Autodesk Inventor part; units mm, degrees
(part 2 of 2)
  arc A490 (63.341, 28.73) -> (62.579, 28.73) centre (62.96, 28.73) ccw
  arc A491 (65.119, 28.73) -> (65.881, 28.73) centre (65.5, 28.73) ccw
  arc A492 (65.881, 28.73) -> (65.119, 28.73) centre (65.5, 28.73) ccw
  arc A493 (65.119, 28.73) -> (65.881, 28.73) centre (65.5, 28.73) ccw
  arc A494 (65.881, 28.73) -> (65.119, 28.73) centre (65.5, 28.73) ccw
  arc A495 (67.659, 28.73) -> (68.421, 28.73) centre (68.04, 28.73) ccw
  arc A496 (68.421, 28.73) -> (67.659, 28.73) centre (68.04, 28.73) ccw
  arc A497 (67.659, 28.73) -> (68.421, 28.73) centre (68.04, 28.73) ccw
  arc A498 (68.421, 28.73) -> (67.659, 28.73) centre (68.04, 28.73) ccw
  arc A499 (70.199, 28.73) -> (70.961, 28.73) centre (70.58, 28.73) ccw
  arc A500 (70.961, 28.73) -> (70.199, 28.73) centre (70.58, 28.73) ccw
  arc A501 (70.199, 28.73) -> (70.961, 28.73) centre (70.58, 28.73) ccw
  arc A502 (70.961, 28.73) -> (70.199, 28.73) centre (70.58, 28.73) ccw
  arc A503 (72.739, 28.73) -> (73.501, 28.73) centre (73.12, 28.73) ccw
  arc A504 (73.501, 28.73) -> (72.739, 28.73) centre (73.12, 28.73) ccw
  arc A505 (72.739, 28.73) -> (73.501, 28.73) centre (73.12, 28.73) ccw
  arc A506 (73.501, 28.73) -> (72.739, 28.73) centre (73.12, 28.73) ccw
  arc A507 (75.279, 28.73) -> (76.041, 28.73) centre (75.66, 28.73) ccw
  arc A508 (76.041, 28.73) -> (75.279, 28.73) centre (75.66, 28.73) ccw
  arc A509 (75.279, 28.73) -> (76.041, 28.73) centre (75.66, 28.73) ccw
  arc A510 (76.041, 28.73) -> (75.279, 28.73) centre (75.66, 28.73) ccw
  arc A511 (77.819, 28.73) -> (78.581, 28.73) centre (78.2, 28.73) ccw
  arc A512 (78.581, 28.73) -> (77.819, 28.73) centre (78.2, 28.73) ccw
  arc A513 (77.819, 28.73) -> (78.581, 28.73) centre (78.2, 28.73) ccw
  arc A514 (78.581, 28.73) -> (77.819, 28.73) centre (78.2, 28.73) ccw
  arc A515 (89.59, 30.6) -> (89.59, 29.7) centre (89.59, 30.15) ccw
  arc A516 (89.59, 29.7) -> (89.59, 30.6) centre (89.59, 30.15) ccw
  arc A517 (89.59, 30.6) -> (89.59, 29.7) centre (89.59, 30.15) ccw
  arc A518 (89.59, 29.7) -> (89.59, 30.6) centre (89.59, 30.15) ccw
  arc A519 (87.05, 30.6) -> (87.05, 29.7) centre (87.05, 30.15) ccw
  arc A520 (87.05, 29.7) -> (87.05, 30.6) centre (87.05, 30.15) ccw
  arc A521 (87.05, 30.6) -> (87.05, 29.7) centre (87.05, 30.15) ccw
  arc A522 (87.05, 29.7) -> (87.05, 30.6) centre (87.05, 30.15) ccw
  arc A523 (84.51, 30.6) -> (84.51, 29.7) centre (84.51, 30.15) ccw
  arc A524 (84.51, 29.7) -> (84.51, 30.6) centre (84.51, 30.15) ccw
  arc A525 (84.51, 30.6) -> (84.51, 29.7) centre (84.51, 30.15) ccw
  arc A526 (84.51, 29.7) -> (84.51, 30.6) centre (84.51, 30.15) ccw
  line L251 (44.7388, 33.8709) -> (94, 33.8709)
  line L252 (94, 33.8709) -> (94, 24.2027)
  line L253 (94, 24.2027) -> (44.7388, 24.2027)
  line L254 (44.7388, 24.2027) -> (44.7388, 33.8709)
  line L255 (28.3727, 38.1472) -> (43.5417, 38.1472)
  line L256 (43.5417, 38.1472) -> (43.5417, 25.8726)
  line L257 (43.5417, 25.8726) -> (28.3727, 25.8726)
  line L258 (28.3727, 25.8726) -> (28.3727, 38.1472)
  line L259 (0, 194.7239) -> (130, 194.7239)
  line L260 (130, 194.7239) -> (130, 0)
  line L261 (130, 0) -> (0, 0)
  line L262 (0, 0) -> (0, 194.7239)
  circle A527 centre (65, 97.362) radius 8
  arc A528 (69.6765, 160.0343) -> (60.3235, 160.0343) centre (65, 167.7239) ccw
  line L263 (74.3631, 160.0343) -> (74.3631, 147.2613)
  line L264 (74.3631, 147.2613) -> (42.3354, 147.2613)
  line L265 (42.3354, 147.2613) -> (42.3354, 160.0343)
  line L266 (78, 180.9909) -> (100.5174, 180.9909)
  line L267 (100.5174, 180.9909) -> (100.5174, 168.379)
  line L268 (100.5174, 168.379) -> (78, 168.379)
  line L269 (78, 168.379) -> (78, 180.9909)
  line L270 (28.3727, 38.1472) -> (43.5417, 38.1472)
  line L271 (43.5417, 38.1472) -> (43.5417, 25.8726)
  line L272 (43.5417, 25.8726) -> (28.3727, 25.8726)
  line L273 (28.3727, 25.8726) -> (28.3727, 38.1472)
  line L274 (44.7388, 33.8709) -> (94, 33.8709)
  line L275 (94, 33.8709) -> (94, 24.2027)
  line L276 (94, 24.2027) -> (44.7388, 24.2027)
  line L277 (44.7388, 24.2027) -> (44.7388, 33.8709)
  circle A529 centre (45.5, 82.362) radius 1.6
  circle A530 centre (55.5, 82.362) radius 1.6
  circle A531 centre (65.5, 82.362) radius 1.6
  circle A532 centre (75.5, 82.362) radius 1.6
  circle A533 centre (85.5, 82.362) radius 1.6
  circle A534 centre (95.5, 82.362) radius 1.6
  circle A535 centre (45.5, 52.362) radius 1.6
  circle A536 centre (55.5, 52.362) radius 1.6
  circle A537 centre (65.5, 52.362) radius 1.6
  circle A538 centre (75.5, 52.362) radius 1.6
  circle A539 centre (85.5, 52.362) radius 1.6
  circle A540 centre (95.5, 52.362) radius 1.6
  circle A541 centre (34.5, 112.362) radius 1.6
  circle A542 centre (44.5, 112.362) radius 1.6
  circle A543 centre (54.5, 112.362) radius 1.6
  circle A544 centre (64.5, 112.362) radius 1.6
  circle A545 centre (74.5, 112.362) radius 1.6
  circle A546 centre (84.5, 112.362) radius 1.6
  circle A547 centre (34.5, 142.362) radius 1.6
  circle A548 centre (44.5, 142.362) radius 1.6
  circle A549 centre (54.5, 142.362) radius 1.6
  circle A550 centre (64.5, 142.362) radius 1.6
  circle A551 centre (74.5, 142.362) radius 1.6
  circle A552 centre (84.5, 142.362) radius 1.6
  circle A553 centre (38, 186.7239) radius 2.15
  circle A554 centre (52, 186.7239) radius 2.15
  circle A555 centre (78, 186.7239) radius 2.15
  circle A556 centre (92, 186.7239) radius 2.15
  circle A557 centre (38, 8) radius 2.15
  circle A558 centre (52, 8) radius 2.15
  circle A559 centre (78, 8) radius 2.15
  circle A560 centre (92, 8) radius 2.15
  circle A561 centre (8, 186.7239) radius 1.6
  circle A562 centre (122, 186.7239) radius 1.6
  circle A563 centre (122, 147.7239) radius 1.6
  circle A564 centre (122, 8) radius 1.6
  circle A565 centre (8, 8) radius 1.6
  line L278 (42.3354, 160.0343) -> (60.3235, 160.0343)
  line L279 (69.6765, 160.0343) -> (74.3631, 160.0343)
  point P0 (0, 0)
  constraints: 980 point on circle, 566 centre point, 560 end point, 40 coincident, 37 concentric, 20 parallel, 11 horizontal, 11 perpendicular, 2 point on line
sketch "スケッチ2" plane through (0, 0, 0) normal (0, 0, 1) x (1, 0, 0)
  point P0 (0, 0)
extrude "押し出し1" add sketch "スケッチ1" along normal blind 5.5 contours L3 L5 A32 L4 A17 A11 L251 L254 L253 L0 | L4 L253 L252 L251 A11 A17 A32 L5 L1 L0 | L3 L2 L4 A33 L58 L53 L52 A23 A29 A32 L5 | L5 A32 L4 A29 A23 L52 L51 L59 A33 L2 L1
